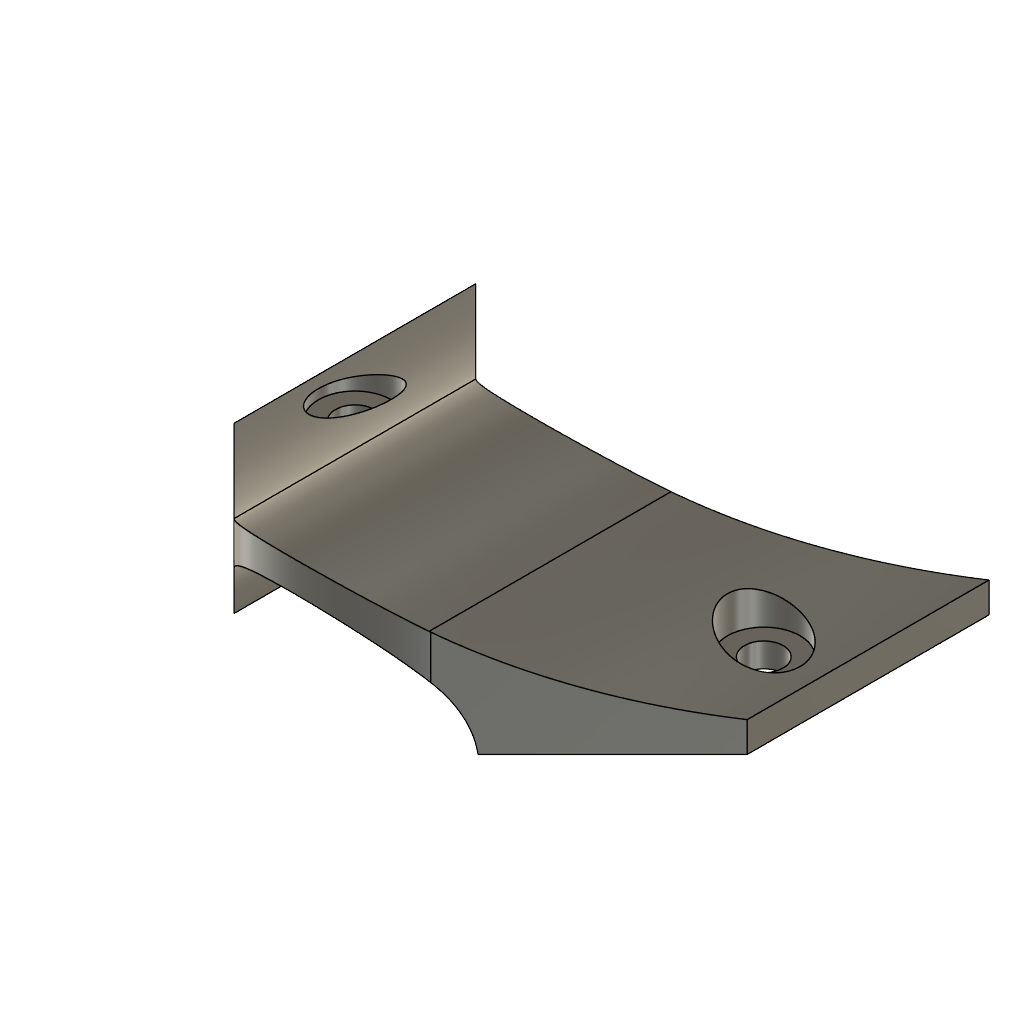
plate+mount (Autodesk Fusion 360 design; units mm, degrees)
part number: 2026-09-13-19-33-41-246
Autodesk Fusion 360 part; units mm, degrees
sketch "Sketch1" plane through (0, 0, 0) normal (0, 0, 1) x (1, 0, 0)
  line L0 (0, 0) -> (21.2132, 21.2132)
  line L1 (0, 0) -> (30, 0) construction
  line L2 (0, 0) -> (-21.2132, 21.2132)
  line L3 (0, 0) -> (30, 0) construction
  line L4 (21.2132, 21.2132) -> (21.2132, 41.2132)
  line L5 (-21.2132, 21.2132) -> (-21.2132, 41.2132)
  line L6 (-21.2132, 41.2132) -> (0, 20)
  line L7 (0, 20) -> (21.2132, 41.2132)
  line L8 (0, 0) -> (10.125, 0)
  line L9 (10.125, 0) -> (10.125, 30.125)
  line L10 (0, 0) -> (-10.125, 0)
  line L11 (-10.125, 0) -> (-10.125, 30.125)
  line L12 (-10.125, 30.125) -> (10.125, 30.125)
  dimension "d1" = 30
  dimension "d2" = 45
  dimension "d3" = 135
  dimension "d4" = 30
  dimension "d5" = 20
  dimension "d6" = 20
  dimension "d7" = 10.125
  dimension "d8" = 10.125
  constraint horizontal L1
  constraint coincident L0.start L1.start
  constraint horizontal L3
  constraint vertical L4
  constraint vertical L5
  constraint perpendicular L6 L7
  constraint coincident L1.end L3.end
  constraint parallel L2 L6
  constraint equal L0 L1
  constraint parallel L3 L8
  constraint coincident L7 L9.end
  constraint perpendicular L8 L9
  constraint perpendicular L9 L10
  constraint coincident L6 L11.end
  constraint perpendicular L10 L11
  measures "d1" distance of L0.start L0.end
  measures "d2" angle of L0 L1
  measures "d3" angle of L2 L3
  measures "d4" distance of L0.start L2.end
  measures "d5" distance of L0.end L4.end
  measures "d6" distance of L2.end L5.end
  measures "d7" distance of L0.start L8.end
  measures "d8" distance of L0.start L10.end
sketch "Sketch2" plane through (0, 0, 0) normal (0, 1, 0) x (1, 0, 0)
  circle A0 centre (0, 0) radius 10.125
  line L0 (0, 0) -> (10.0865, -0.8825)
  line L1 (0, 0) -> (9.6779, 0) construction
  line L2 (0, 0) -> (-10.0865, -0.8825)
  line L3 (0, 0) -> (10.125, 0) construction
  line L4 (-10.0865, -0.8825) -> (10.0865, -0.8825)
  line L5 (10.0865, -0.8825) -> (12.5865, -0.8825)
  circle A1 centre (0, 0) radius 12.6174
  line L6 (-10.0865, -0.8825) -> (-12.5865, -0.8825)
  dimension "d9" = 20.25
  dimension "d10" = 5
  dimension "d11" = 175
  dimension "d13" = 2.5
  dimension "d18" = 9.6779
  constraint coincident A0.centre L0.start
  constraint horizontal L1
  constraint coincident A0 L0.end
  constraint horizontal L3
  constraint coincident A0 L2.end
  constraint parallel L4 L5
  constraint concentric A0 A1
  constraint coincident L5.end A1
  constraint coincident A1 L6.end
  constraint parallel L4 L6
  constraint coincident A0 L3.end
  measures "d9" diameter of A0
  measures "d10" angle of L0 L1
  measures "d11" angle of L2 L3
  measures "d13" distance of L0.end L5.end
  measures "d18" horizontal distance of A0.centre L1.end
ref_plane "WorkPlane1" through (0, 0, 0.8825) normal (0, 0, 1) x (1, 0, 0)
sketch "Sketch3" plane through (0, 0, 0.8825) normal (0, 0, 1) x (1, 0, 0)
  line L0 (-10.0865, 0) -> (10.0865, 0)
  line L1 (0, 0) -> (-21.2132, 21.2132)
  line L2 (-21.2132, 21.2132) -> (-21.2132, 41.2132)
  line L3 (-21.2132, 41.2132) -> (0, 20)
  line L4 (0, 20) -> (21.2132, 41.2132)
  line L5 (0, 0) -> (21.2132, 21.2132)
  line L6 (21.2132, 21.2132) -> (21.2132, 41.2132)
  line L7 (0, 0) -> (-21.2132, 21.2132)
  line L8 (-21.2132, 21.2132) -> (-21.2132, 41.2132)
  line L9 (-21.2132, 41.2132) -> (0, 20)
  line L10 (0, 20) -> (21.2132, 41.2132)
  line L11 (21.2132, 41.2132) -> (21.2132, 21.2132)
  line L12 (21.2132, 21.2132) -> (0, 0)
  line L13 (-10.0865, 0) -> (-10.0865, 30.0865)
  line L14 (10.0865, 0) -> (10.0865, 30.0865)
  line L15 (10.0865, 30.0865) -> (-10.0865, 30.0865)
  line L16 (10.0865, 0) -> (0, 0)
  line L17 (0, 0) -> (-10.0865, 0)
  line L18 (10.0865, 0) -> (12.5865, 0)
  line L19 (12.5865, 0) -> (12.5865, 32.5865)
  line L20 (12.5865, 32.5865) -> (-12.5865, 32.5865)
  line L21 (-10.0865, 0) -> (-12.5865, 0)
  line L22 (-12.5865, 0) -> (-12.5865, 32.5865)
  line L23 (-12.5865, 22.5865) -> (-21.2132, 31.2132) construction
  line L24 (-16.8998, 26.8998) -> (-16.8998, 16.8998) construction
  line L25 (-16.8998, 26.8998) -> (-16.8998, 36.8998) construction
  circle A0 centre (-16.8998, 26.8998) radius 1.6
  circle A1 centre (-16.8998, 26.8998) radius 3
  dimension "d16" = 2.5
  dimension "d17" = 2.5
  dimension "d35" = 3.2
  dimension "d38" = 6
  constraint coincident L1.start L5.start
  constraint coincident L1.end L2.start
  constraint coincident L2.end L3.start
  constraint coincident L3.end L4.start
  constraint coincident L4.end L6.end
  constraint coincident L5.end L6.start
  constraint coincident L0.start L13.start
  constraint coincident L3 L13.end
  constraint perpendicular L0 L13
  constraint coincident L0.end L14.start
  constraint coincident L4 L14.end
  constraint perpendicular L0 L14
  constraint perpendicular L14 L18
  constraint coincident L10 L19.end
  constraint perpendicular L18 L19
  constraint coincident L9 L20.end
  constraint perpendicular L19 L20
  constraint perpendicular L13 L21
  constraint coincident L22 L23.start
  constraint midpoint L2 L23.end
  constraint parallel L9 L23
  constraint midpoint L23 L24.start
  constraint coincident L7 L24.end
  constraint vertical L24
  constraint coincident L3 L25.end
  constraint parallel L24 L25
  constraint coincident L24.start L25.start
  constraint concentric A0 A1
  measures "d16" distance of L0.end L18.end
  measures "d17" distance of L0.start L21.end
  measures "d35" diameter of A0
  measures "d38" diameter of A1
extrude "Extrude1" add sketch "Sketch3" along normal blind 2.5 contours L1 L3 L4 L5 L7 L9 L10 L12 L13 L14 | L1 L3 L7 L9 L13 L22 | L4 L5 L10 L12 L14 L19 | L1 L2 L3 L7 L8 L9 L22 | L4 L5 L6 L10 L11 L12 L19 | A0 | A1
extrude "Extrude2" add sketch "Sketch2" along normal blind 32.586 contours A0 L5 A1 L6 picked at (0, -11.7651)
extrude "Extrude3" cut sketch "Sketch3" along normal blind 18 contours L3 L4 L9 L10 L15 | L3 L4 L9 L10 L15 L20
sketch "Sketch4" plane through (0, 0, 0) normal (0, 1, 0) x (1, 0, 0)
  arc A0 (-10.0865, -0.8825) -> (-9.5433, -3.3825) centre (0, 0) ccw
  line L0 (-10.0865, -0.8825) -> (0, -0.8825)
  line L1 (0, -0.8825) -> (0, -3.3825)
  line L2 (0, -3.3825) -> (-9.5433, -3.3825)
  arc A1 (9.5433, -3.3825) -> (10.0865, -0.8825) centre (0, 0) ccw
  line L3 (9.5433, -3.3825) -> (0, -3.3825)
  line L4 (0, -3.3825) -> (0, -0.8825)
  line L5 (0, -0.8825) -> (10.0865, -0.8825)
extrude "Extrude4" cut sketch "Sketch4" along normal blind 59
extrude "Extrude5" cut sketch "Sketch3" along normal blind 16 contours L0 L1 L7 L13 L17 | L1 L7 L13 L21 L22 | L0 L5 L12 L14 L16 | L5 L12 L14 L18 L19
fillet "Fillet1" radius 30 2 edges at (12.1555, 22.1555, 3.3825) (-12.1555, 22.1555, 3.3825)
fillet "Fillet1" radius 11.5 1 edges at (0, 20, 11.3712)
fillet "Fillet2" radius 11.5 1 edges at (0, 0, 11.3712)
extrude "Extrude6" cut sketch "Sketch3" along normal blind 5 contours A0
extrude "Extrude7" cut sketch "Sketch3" along normal blind 4 from surface at 2 contours A1
ref_plane "WorkPlane2" through (0, 31.2132, 2.1325) normal (-1, 0, 0) x (0, -1, 0)
mirror "Mirror1" about plane through (0, 31.2132, 2.1325) normal (-1, 0, 0) of "Extrude6", "Extrude7"
